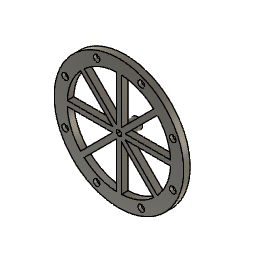
Circle Out V2 v1 (Autodesk Fusion 360 design; units mm, degrees)
Autodesk Fusion 360 part; units mm, degrees
sketch "Sketch1" plane through (0, 0, 0) normal (0, 1, 0) x (1, 0, 0) in component "Circle Out"
  circle A0 centre (0, 0) radius 50
  circle A1 centre (0, 0) radius 40
  circle A2 centre (0, 0) radius 4.5
  line L0 (11.5858, -14.4142) -> (2, -4.8284)
  line L1 (2, -20) -> (2, -39.95)
  line L2 (11.5858, -14.4142) -> (26.8347, -29.6631)
  line L3 (-2, -20) -> (-2, -39.95)
  line L4 (14.4142, -11.5858) -> (29.6631, -26.8347)
  line L5 (24, -2) -> (4.8284, -2)
  line L6 (24, -2) -> (39.95, -2)
  line L7 (24, 2) -> (39.95, 2)
  line L8 (16.7362, 13.9078) -> (4.8284, 2)
  line L9 (16.7362, 13.9078) -> (29.6631, 26.8347)
  line L10 (13.9078, 16.7362) -> (26.8347, 29.6631)
  line L11 (2, 15) -> (2, 4.8284)
  line L12 (2, 15) -> (2, 39.95)
  line L13 (-2, 15) -> (-2, 39.95)
  line L14 (-8.5858, 11.4142) -> (-2, 4.8284)
  line L15 (-8.5858, 11.4142) -> (-26.8347, 29.6631)
  line L16 (-11.4142, 8.5858) -> (-11.591, 8.7626)
  line L17 (-11.591, 8.7626) -> (-29.6631, 26.8347)
  line L18 (-14, 2) -> (-4.8284, 2)
  line L19 (-14, 2) -> (-39.95, 2)
  line L20 (-14, -2) -> (-39.95, -2)
  line L21 (-13.0052, -10.1768) -> (-4.8284, -2)
  line L22 (-13.0052, -10.1768) -> (-29.6631, -26.8347)
  line L23 (-10.1768, -13.0052) -> (-26.8347, -29.6631)
  line L24 (-10.1768, -13.0052) -> (-2, -4.8284)
  line L25 (-2, -4.8284) -> (-2, -39.95)
  line L26 (2, -4.8284) -> (2, -20)
  line L27 (4.8284, -2) -> (14.4142, -11.5858)
  line L28 (4.8284, 2) -> (24, 2)
  line L29 (2, 4.8284) -> (13.9078, 16.7362)
  line L30 (-2, 4.8284) -> (-2, 15)
  line L31 (-4.8284, 2) -> (-11.4142, 8.5858)
  line L32 (-14, -2) -> (-4.8284, -2)
  dimension "d2" = 100
  dimension "d3" = 9
  constraint coincident A0.centre A1.centre
  constraint concentric A0 A2
  constraint coincident A1 L1.end
  constraint coincident A1 L2.end
  constraint coincident A1 L3.end
  constraint coincident A1 L4.end
  constraint coincident A1 L6.end
  constraint coincident A1 L7.end
  constraint coincident A1 L9.end
  constraint coincident A1 L10.end
  constraint coincident A1 L12.end
  constraint coincident A1 L13.end
  constraint coincident A1 L15.end
  constraint coincident A1 L17.end
  constraint coincident A1 L19.end
  constraint coincident A1 L20.end
  constraint coincident A1 L22.end
  constraint coincident A1 L23.end
  constraint parallel L3 L25
  constraint parallel L1 L26
  constraint parallel L4 L27
  constraint parallel L7 L28
  constraint parallel L10 L29
  constraint perpendicular L20 L30
  constraint parallel L16 L31
  constraint horizontal L32
  measures "d2" diameter of A0
  measures "d3" diameter of A2
extrude "Extrude1" add sketch "Sketch1" along normal blind 5 contours A0 | A1 L0 L1 L2 L3 L4 L5 L6 L7 L8 L9 L10 L11 L12 L13 L14 L15 L16 L17 L18 L19 L20 L21 L22 L23 L24 L25 L26 L27 L28 L29 L30 L31 L32 | A2 in component "Circle Out"
sketch "Sketch2" plane through (0, 5, 0) normal (0, 1, 0) x (-1, 0, 0) in component "Circle Out"
  line L0 (4.8284, -2) -> (39.95, -2)
  arc A0 (29.6631, -26.8347) -> (39.95, -2) centre (0, 0) ccw
  line L1 (29.6631, -26.8347) -> (4.8284, -2)
  line L2 (-2, -4.8284) -> (-2, -39.95)
  arc A1 (-26.8347, -29.6631) -> (-2, -39.95) centre (0, 0) ccw
  line L3 (-26.8347, -29.6631) -> (-2, -4.8284)
  line L4 (2, -4.8284) -> (26.8347, -29.6631)
  arc A2 (2, -39.95) -> (26.8347, -29.6631) centre (0, 0) ccw
  line L5 (2, -39.95) -> (2, -4.8284)
  line L6 (-4.8284, -2) -> (-29.6631, -26.8347)
  arc A3 (-39.95, -2) -> (-29.6631, -26.8347) centre (0, 0) ccw
  line L7 (-39.95, -2) -> (-4.8284, -2)
  arc A4 (39.95, 2) -> (29.6631, 26.8347) centre (0, 0) ccw
  line L8 (39.95, 2) -> (4.8284, 2)
  line L9 (4.8284, 2) -> (29.6631, 26.8347)
  line L10 (-4.8284, 2) -> (-39.95, 2)
  arc A5 (-29.6631, 26.8347) -> (-39.95, 2) centre (0, 0) ccw
  line L11 (-29.6631, 26.8347) -> (-4.8284, 2)
  line L12 (26.8347, 29.6631) -> (2, 4.8284)
  line L13 (2, 4.8284) -> (2, 39.95)
  arc A6 (26.8347, 29.6631) -> (2, 39.95) centre (0, 0) ccw
  line L14 (-2, 4.8284) -> (-26.8347, 29.6631)
  arc A7 (-2, 39.95) -> (-26.8347, 29.6631) centre (0, 0) ccw
  line L15 (-2, 39.95) -> (-2, 4.8284)
  circle A8 centre (0, 0) radius 50
  circle A9 centre (0, 0) radius 4.25
  dimension "d25" = 8.5
  constraint concentric A0 A9
  measures "d25" diameter of A9
extrude "Extrude2" add sketch "Sketch2" along normal blind 9 contours A9 in component "Circle Out"
sketch "Sketch3" plane through (0, 14, 0) normal (0, 1, 0) x (-1, 0, 0) in component "Circle Out"
  circle A0 centre (0, 0) radius 4.25
  line L0 (-2, 0) -> (-2, 1.3)
  line L1 (-2, 1.3) -> (0, 2)
  line L2 (2, 0) -> (2, 1.3)
  line L3 (2, 1.3) -> (0, 2)
  line L4 (-2, 0) -> (-2, -1.3)
  line L5 (-2, -1.3) -> (0, -2)
  line L6 (2, 0) -> (2, -1.3)
  line L7 (2, -1.3) -> (0, -2)
  constraint parallel L3 L5
extrude "Extrude3" cut sketch "Sketch3" against normal blind 16 contours L0 L1 L2 L3 L4 L5 L6 L7 in component "Circle Out"
sketch "Sketch4" plane through (0, 0, 0) normal (0, -1, 0) x (1, 0, 0) in component "Circle Out"
  line L0 (-2, 1.3) -> (0, 2)
  line L1 (0, 2) -> (2, 1.3)
  line L2 (2, 1.3) -> (2, -1.3)
  line L3 (2, -1.3) -> (0, -2)
  line L4 (0, -2) -> (-2, -1.3)
  line L5 (-2, -1.3) -> (-2, 1.3)
  line L6 (-39.95, -2) -> (-4.8284, -2)
  line L7 (-4.8284, -2) -> (-29.6631, -26.8347)
  arc A0 (-39.95, -2) -> (-29.6631, -26.8347) centre (0, 0) ccw
  line L8 (2, -39.95) -> (2, -4.8284)
  line L9 (2, -4.8284) -> (26.8347, -29.6631)
  arc A1 (2, -39.95) -> (26.8347, -29.6631) centre (0, 0) ccw
  line L10 (-26.8347, -29.6631) -> (-2, -4.8284)
  line L11 (-2, -4.8284) -> (-2, -39.95)
  arc A2 (-26.8347, -29.6631) -> (-2, -39.95) centre (0, 0) ccw
  line L12 (29.6631, -26.8347) -> (4.8284, -2)
  line L13 (4.8284, -2) -> (39.95, -2)
  arc A3 (29.6631, -26.8347) -> (39.95, -2) centre (0, 0) ccw
  arc A4 (-29.6631, 26.8347) -> (-39.95, 2) centre (0, 0) ccw
  line L14 (-29.6631, 26.8347) -> (-4.8284, 2)
  line L15 (-4.8284, 2) -> (-39.95, 2)
  line L16 (39.95, 2) -> (4.8284, 2)
  line L17 (4.8284, 2) -> (29.6631, 26.8347)
  arc A5 (39.95, 2) -> (29.6631, 26.8347) centre (0, 0) ccw
  line L18 (-2, 4.8284) -> (-26.8347, 29.6631)
  arc A6 (-2, 39.95) -> (-26.8347, 29.6631) centre (0, 0) ccw
  line L19 (-2, 39.95) -> (-2, 4.8284)
  line L20 (26.8347, 29.6631) -> (2, 4.8284)
  line L21 (2, 4.8284) -> (2, 39.95)
  arc A7 (26.8347, 29.6631) -> (2, 39.95) centre (0, 0) ccw
  circle A8 centre (0, 0) radius 50
  circle A9 centre (-17.2208, 41.5746) radius 2.5
  circle A10 centre (-41.5746, 17.2208) radius 2.5
  circle A11 centre (-41.5746, -17.2208) radius 2.5
  circle A12 centre (-17.2208, -41.5746) radius 2.5
  circle A13 centre (17.2208, -41.5746) radius 2.5
  circle A14 centre (41.5746, -17.2208) radius 2.5
  circle A15 centre (41.5746, 17.2208) radius 2.5
  circle A16 centre (17.2208, 41.5746) radius 2.5
  dimension "d32" = 5
  dimension "d33" = 5
  dimension "d34" = 5
  dimension "d35" = 5
  dimension "d36" = 5
  dimension "d37" = 5
  dimension "d38" = 5
  dimension "d39" = 5
  measures "d32" diameter of A9
  measures "d33" diameter of A10
  measures "d34" diameter of A11
  measures "d35" diameter of A12
  measures "d36" diameter of A13
  measures "d37" diameter of A14
  measures "d38" diameter of A15
  measures "d39" diameter of A16
extrude "Extrude4" cut sketch "Sketch4" against normal blind 10 contours A9 | A10 | A11 | A12 | A13 | A14 | A15 | A16 in component "Circle Out"
sketch "Sketch5" plane through (0, 5, 0) normal (0, 1, 0) x (-1, 0, 0) in component "Circle Out"
  circle A0 centre (-41.5746, 17.2208) radius 2.5
  circle A1 centre (41.5746, -17.2208) radius 2.5
  circle A2 centre (17.2208, -41.5746) radius 2.5
  circle A3 centre (-17.2208, 41.5746) radius 2.5
  circle A4 centre (-41.5746, -17.2208) radius 2.5
  circle A5 centre (41.5746, 17.2208) radius 2.5
  circle A6 centre (-17.2208, -41.5746) radius 2.5
  circle A7 centre (17.2208, 41.5746) radius 2.5
  circle A8 centre (0, 0) radius 4.25
  line L0 (4.8284, -2) -> (39.95, -2)
  arc A9 (29.6631, -26.8347) -> (39.95, -2) centre (0, 0) ccw
  line L1 (29.6631, -26.8347) -> (4.8284, -2)
  line L2 (-2, -4.8284) -> (-2, -39.95)
  arc A10 (-26.8347, -29.6631) -> (-2, -39.95) centre (0, 0) ccw
  line L3 (-26.8347, -29.6631) -> (-2, -4.8284)
  line L4 (2, -4.8284) -> (26.8347, -29.6631)
  arc A11 (2, -39.95) -> (26.8347, -29.6631) centre (0, 0) ccw
  line L5 (2, -39.95) -> (2, -4.8284)
  line L6 (-4.8284, -2) -> (-29.6631, -26.8347)
  arc A12 (-39.95, -2) -> (-29.6631, -26.8347) centre (0, 0) ccw
  line L7 (-39.95, -2) -> (-4.8284, -2)
  arc A13 (39.95, 2) -> (29.6631, 26.8347) centre (0, 0) ccw
  line L8 (39.95, 2) -> (4.8284, 2)
  line L9 (4.8284, 2) -> (29.6631, 26.8347)
  line L10 (-4.8284, 2) -> (-39.95, 2)
  arc A14 (-29.6631, 26.8347) -> (-39.95, 2) centre (0, 0) ccw
  line L11 (-29.6631, 26.8347) -> (-4.8284, 2)
  line L12 (26.8347, 29.6631) -> (2, 4.8284)
  line L13 (2, 4.8284) -> (2, 39.95)
  arc A15 (26.8347, 29.6631) -> (2, 39.95) centre (0, 0) ccw
  line L14 (-2, 4.8284) -> (-26.8347, 29.6631)
  arc A16 (-2, 39.95) -> (-26.8347, 29.6631) centre (0, 0) ccw
  line L15 (-2, 39.95) -> (-2, 4.8284)
  circle A17 centre (0, 0) radius 50
  circle A18 centre (-17.2208, 41.5746) radius 4.25
  circle A19 centre (17.2208, 41.5746) radius 4.25
  circle A20 centre (-41.5746, 17.2208) radius 4.25
  circle A21 centre (-41.5746, -17.2208) radius 4.25
  circle A22 centre (-17.2208, -41.5746) radius 4.25
  circle A23 centre (17.2208, -41.5746) radius 4.25
  circle A24 centre (41.5746, -17.2208) radius 4.25
  circle A25 centre (41.5746, 17.2208) radius 4.25
  dimension "d42" = 8.5
  dimension "d43" = 8.5
  dimension "d44" = 8.5
  dimension "d45" = 8.5
  dimension "d46" = 8.5
  dimension "d47" = 8.5
  dimension "d48" = 8.5
  dimension "d49" = 8.5
  constraint concentric A3 A18
  constraint concentric A7 A19
  constraint concentric A0 A20
  constraint concentric A4 A21
  constraint concentric A6 A22
  constraint concentric A2 A23
  constraint concentric A1 A24
  constraint concentric A5 A25
  measures "d42" diameter of A18
  measures "d43" diameter of A19
  measures "d44" diameter of A20
  measures "d45" diameter of A21
  measures "d46" diameter of A22
  measures "d47" diameter of A23
  measures "d48" diameter of A24
  measures "d49" diameter of A25
extrude "Extrude5" cut sketch "Sketch5" against normal blind 2.5 contours A18 | A19 | A20 | A21 | A22 | A23 | A24 | A25 in component "Circle Out"
component "Circle Out" placed x (1, 0, 0) y (0, 1, 0) z (0, 0, 1) at (0, 0, 0)
